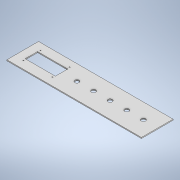
# Autodesk Inventor part: 220307 Lid Part B
Saved by Autodesk Inventor 2022 (Build 260153000, 153)
## iProperties
Created: 2022-02-07
Part Number: 220307 Lid Part B
Material: Generic
Document SubType Name: Modeling
Designer: josephinew
Density: 1 g/cm^3
Appearance: Default
Author: josephinew
Autodesk Inventor part; units mm, degrees
ref_plane "YZ Plane" through (0, 0, 0) normal (1, 0, 0) x (0, 1, 0)
ref_plane "XZ Plane" through (0, 0, 0) normal (0, 1, 0) x (-1, 0, 0)
ref_plane "XY Plane" through (0, 0, 0) normal (0, 0, 1) x (1, 0, 0)
sketch "Sketch1" plane through (0, 0, 0) normal (0, 1, 0) x (-1, 0, 0)
  line L0 (0, 0) -> (-431.8, 0)
  line L1 (-431.8, 0) -> (-431.8, -431.8)
  line L2 (-431.8, -431.8) -> (0, -431.8)
  line L3 (0, -431.8) -> (0, 0)
  dimension "d0" = 431.8
  dimension "d1" = 431.8
  constraints: 8 end point, 2 parallel, 1 horizontal, 1 perpendicular
  measures "d0" distance of L2.end L1.end
  measures "d1" distance of L1.end L0.end
extrude "Extrusion1" add sketch "Sketch1" along normal blind 3.175
sketch "Sketch2" plane through (0, 3.175, 0) normal (0, 1, 0) x (1, 0, 0)
  line L0 (0, 431.8) -> (0, 0) projected
  line L1 (431.8, 0) -> (431.8, 431.8) projected
  circle A0 centre (386.08, 64.77) radius 6.35
  circle A1 centre (332.74, 64.77) radius 6.35
  circle A2 centre (279.4, 64.77) radius 6.35
  circle A3 centre (226.06, 64.77) radius 6.35
  circle A4 centre (172.72, 64.77) radius 6.35
  circle A5 centre (28.43, 92.2674) radius 1.5
  circle A6 centre (121.43, 92.2674) radius 1.5
  circle A7 centre (28.43, 37.2726) radius 1.5
  circle A8 centre (121.43, 37.2726) radius 1.5
  line L2 (26.43, 84.77) -> (123.43, 84.77)
  line L3 (123.43, 84.77) -> (123.43, 44.77)
  line L4 (123.43, 44.77) -> (26.43, 44.77)
  line L5 (26.43, 44.77) -> (26.43, 84.77)
  dimension "d14" = 12.7
  dimension "d15" = 12.7
  dimension "d16" = 12.7
  dimension "d17" = 12.7
  dimension "d18" = 12.7
  constraints: 9 centre point, 8 end point, 2 parallel, 1 horizontal, 1 perpendicular
  measures "d14" diameter of A0
  measures "d15" diameter of A1
  measures "d16" diameter of A2
  measures "d17" diameter of A3
  measures "d18" diameter of A4
extrude "Extrusion2" cut sketch "Sketch2" against normal blind 25.4
sketch "Sketch3" plane through (0, 3.175, 0) normal (0, 1, 0) x (1, 0, 0)
  line L0 (0, 431.8) -> (0, 0) projected
  line L1 (431.8, 0) -> (431.8, 431.8) projected
  circle A0 centre (88.9, 424.18) radius 2.54
  circle A1 centre (115.316, 424.18) radius 2.54
  circle A2 centre (316.484, 424.18) radius 2.54
  circle A3 centre (342.9, 424.18) radius 2.54
  line L2 (431.8, 431.8) -> (431.8, 424.18)
  constraints: 4 centre point, 2 end point, 1 point on line
extrude "Extrusion3" cut sketch "Sketch3" along normal blind 25.4 and the other way blind 12.7
sketch "Sketch4" plane through (0, 0, 0) normal (0, -1, 0) x (1, 0, 0)
  circle A0 centre (386.08, -64.77) radius 6.35 projected
  circle A1 centre (386.08, -64.77) radius 6.858
  circle A2 centre (172.72, -64.77) radius 6.35 projected
  circle A3 centre (172.72, -64.77) radius 6.858
  circle A4 centre (226.06, -64.77) radius 6.35 projected
  circle A5 centre (226.06, -64.77) radius 6.858
  circle A6 centre (279.4, -64.77) radius 6.35 projected
  circle A7 centre (279.4, -64.77) radius 6.858
  circle A8 centre (332.74, -64.77) radius 6.35 projected
  circle A9 centre (332.74, -64.77) radius 6.858
  point P0 (0, 0)
  dimension "d50" = 13.716
  dimension "d51" = 13.716
  dimension "d52" = 13.716
  dimension "d53" = 13.716
  dimension "d54" = 13.716
  constraints: 5 centre point, 5 coincident
  measures "d50" diameter of A1
  measures "d51" diameter of A3
  measures "d52" diameter of A5
  measures "d53" diameter of A7
  measures "d54" diameter of A9
extrude "Extrusion4" cut sketch "Sketch4" against normal blind 4.351 contours A0 | A1 | A2 | A3 | A4 | A5 | A6 | A7 | A8 | A9
sketch "Sketch6" plane through (0, 3.175, 0) normal (0, 1, 0) x (1, 0, 0)
  line L0 (431.8, 0) -> (431.8, 431.8) projected
  line L1 (0, 431.8) -> (431.8, 431.8)
  line L2 (431.8, 431.8) -> (431.8, 114.3)
  line L3 (431.8, 114.3) -> (0, 114.3)
  line L4 (0, 114.3) -> (0, 431.8)
  line L5 (0, 114.3) -> (431.8, 114.3)
  line L6 (431.8, 114.3) -> (431.8, 12.7)
  line L7 (431.8, 12.7) -> (0, 12.7)
  line L8 (0, 12.7) -> (0, 114.3)
  line L9 (431.8, 0) -> (0, 0)
  line L10 (0, 0) -> (0, 12.7)
  line L11 (0, 12.7) -> (431.8, 12.7)
  line L12 (431.8, 12.7) -> (431.8, 0)
  dimension "d68" = 317.5
  dimension "d69" = 101.6
  constraints: 24 end point, 6 parallel, 3 horizontal, 3 perpendicular, 2 point on line
  measures "d68" distance of L1.end L2.end
  measures "d69" distance of L5.end L6.end
extrude "Extrusion6" cut sketch "Sketch6" against normal blind 25.4 contours L9 L10 L7 L0 | L3 L4 L1 L0
body "Solid1"
